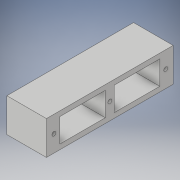
# Autodesk Inventor part: LEG_FEMUR
Saved by Autodesk Inventor 2017 (Build 210142000, 142)
## iProperties
Created: 2017-08-31
Part Number: LEG_FEMUR
Material: Generic
Document SubType Name: Modeling
Designer: Alexander Miller
Density: 1 g/cm^3
Appearance: Default
Author: Alexander Miller
Autodesk Inventor part; units mm, degrees
ref_plane "YZ Plane" through (0, 0, 0) normal (1, 0, 0) x (0, 1, 0)
ref_plane "XZ Plane" through (0, 0, 0) normal (0, 1, 0) x (-1, 0, 0)
ref_plane "XY Plane" through (0, 0, 0) normal (0, 0, 1) x (1, 0, 0)
sketch "Sketch8" plane through (0, 0, 0) normal (0, 1, 0) x (-1, 0, 0)
  line L0 (10, 32) -> (-10, 32)
  line L1 (-10, 32) -> (-10, -32)
  line L2 (-10, -32) -> (10, -32)
  line L3 (10, -32) -> (10, 32)
  point P0 (0, 0)
  point P1 (10, 0)
  point P2 (0, 32)
  dimension "d42" = 20
  dimension "d43" = 64
  constraints: 8 end point, 2 midpoint, 2 parallel, 1 horizontal, 1 horizontal alignment, 1 perpendicular, 1 vertical alignment
  measures "d42" distance of L0.start L0.end
  measures "d43" distance of L2.end L0.start
extrude "Extrusion7" add sketch "Sketch8" along normal blind 17
sketch "Sketch9" plane through (10, 0, 32) normal (1, 0, 0) x (0, 0, -1)
  line L0 (6.75, 14.5) -> (29.75, 14.5)
  line L1 (29.75, 14.5) -> (29.75, 2.5)
  line L2 (29.75, 2.5) -> (6.75, 2.5)
  line L3 (6.75, 2.5) -> (6.75, 14.5)
  line L4 (34.25, 14.5) -> (57.25, 14.5)
  line L5 (57.25, 14.5) -> (57.25, 2.5)
  line L6 (57.25, 2.5) -> (34.25, 2.5)
  line L7 (34.25, 2.5) -> (34.25, 14.5)
  line L8 (0, 0) -> (0, 17) projected
  line L9 (0, 17) -> (64, 17) projected
  line L10 (64, 0) -> (64, 17) projected
  circle A0 centre (3.75, 8.5) radius 1
  circle A1 centre (32, 8.5) radius 1
  circle A2 centre (60.25, 8.5) radius 1
  point P0 (32, 0)
  point P1 (0, 8.5)
  point P2 (6.75, 8.5)
  point P3 (0, 8.5)
  point P4 (32, 17)
  dimension "d46" = 23
  dimension "d47" = 12
  dimension "d48" = 6.75
  dimension "d50" = 6.75
  dimension "d51" = 2
  dimension "d52" = 2
  dimension "d53" = 2
  constraints: 16 end point, 4 horizontal alignment, 4 midpoint, 4 parallel, 3 centre point, 2 equal radius, 2 horizontal, 2 perpendicular, 2 point on line, 1 collinear, 1 vertical alignment
  measures "d46" distance of L0.start L0.end
  measures "d47" distance of L0.end L1.end
  measures "d48" distance between parallel lines of L3 L8
  measures "d50" distance between parallel lines of L10 L5
  measures "d51" diameter of A0
  measures "d52" distance edge to line of A0 L3
  measures "d53" distance edge to line of A2 L5
extrude "Extrusion8" cut sketch "Sketch9" against normal through all
equation "\"d46\" = servo_A"
equation "\"d47\" = servo_B"
equation "\"d50\" = d48"
equation "\"d51\" = servo_H"
equation "\"d52\" = servo_L"
equation "\"d53\" = d52"
equation "\"servo_A\" = 23"
equation "\"servo_B\" = 12"
equation "\"servo_H\" = 2"
equation "\"servo_L\" = 2"
body "Solid4"
